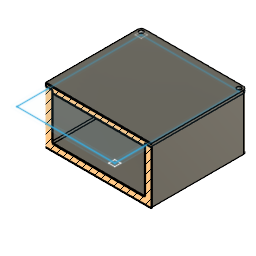
Box (Autodesk Fusion 360 design; units mm, degrees)
part number: 2026-07-20-21-03-58-524
Autodesk Fusion 360 part; units mm, degrees
sketch "Sketch1" plane through (0, 0, 0) normal (0, 0, 1) x (1, 0, 0)
  line L0 (40, -50) -> (-40, -50)
  line L1 (-40, -50) -> (-40, 50)
  line L2 (-40, 50) -> (40, 50)
  line L3 (40, 50) -> (40, -50)
  line L4 (40, -50) -> (-40, 50) construction
  line L5 (-40, -50) -> (40, 50) construction
  dimension "d1" = 80
  dimension "d2" = 100
  constraint horizontal L0
  constraint perpendicular L0 L1
  constraint parallel L0 L2
  constraint parallel L1 L3
  constraint coincident L4 origin
  constraint coincident L5 origin
  measures "d1" distance of L1.end L2.end
  measures "d2" distance of L0.end L1.end
extrude "Extrude1" add sketch "Sketch1" along normal blind 40 makes body 1
shell "Shell1" thickness 5 removed faces 1 at (13.3333, -16.6667, 40) on bodies 1
fillet "Fillet1" radius 2.5 1 edges at (40, -50, 20) on bodies 1
fillet "Fillet2" radius 2.5 1 edges at (40, 50, 20) on bodies 1
fillet "Fillet3" radius 2.5 1 edges at (-40, 50, 20) on bodies 1
fillet "Fillet4" radius 2.5 1 edges at (-40, -50, 20) on bodies 1
fillet "Fillet5" radius 1 8 edges at (-35, -45, 22.5) (0, -45, 5) (-35, 0, 5) (35, -45, 22.5) (35, 0, 5) (35, 45, 22.5) (0, 45, 5) (-35, 45, 22.5) on bodies 1
sketch "Sketch2" plane through (0, 0, 40) normal (0, 0, 1) x (-1, 0, 0)
  arc A0 (40, 47.5) -> (37.5, 50) centre (37.5, 47.5) ccw
  line L0 (37.5, 50) -> (-37.5, 50)
  arc A1 (-37.5, 50) -> (-40, 47.5) centre (-37.5, 47.5) ccw
  line L1 (-40, 47.5) -> (-40, -47.5)
  arc A2 (-40, -47.5) -> (-37.5, -50) centre (-37.5, -47.5) ccw
  line L2 (-37.5, -50) -> (37.5, -50)
  arc A3 (37.5, -50) -> (40, -47.5) centre (37.5, -47.5) ccw
  line L3 (40, -47.5) -> (40, 47.5)
  line L4 (-35, -44) -> (-35, 44)
  arc A4 (-34, 45) -> (-35, 44) centre (-34, 44) ccw
  line L5 (-34, 45) -> (34, 45)
  arc A5 (35, 44) -> (34, 45) centre (34, 44) ccw
  line L6 (35, 44) -> (35, -44)
  arc A6 (34, -45) -> (35, -44) centre (34, -44) ccw
  line L7 (34, -45) -> (-34, -45)
  arc A7 (-35, -44) -> (-34, -45) centre (-34, -44) ccw
  line L8 (-39.2678, 49.2678) -> (-34.7071, 49.2678) construction
  line L9 (-34.7071, 49.2678) -> (-34.7071, 44.7071) construction
  line L10 (-34.7071, 44.7071) -> (-39.2678, 44.7071) construction
  line L11 (-39.2678, 44.7071) -> (-39.2678, 49.2678) construction
  line L12 (34.7071, -44.7071) -> (39.2678, -44.7071) construction
  line L13 (39.2678, -44.7071) -> (39.2678, -49.2678) construction
  line L14 (39.2678, -49.2678) -> (34.7071, -49.2678) construction
  line L15 (34.7071, -49.2678) -> (34.7071, -44.7071) construction
  line L16 (36.9874, -46.9874) -> (-36.9874, -46.9874)
  line L17 (-36.9874, -46.9874) -> (-36.9874, 46.9874)
  line L18 (-36.9874, 46.9874) -> (36.9874, 46.9874)
  line L19 (36.9874, 46.9874) -> (36.9874, -46.9874)
  constraint horizontal L8
  constraint vertical L9
  constraint horizontal L10
  constraint vertical L11
  constraint midpoint A4 L9.end
  constraint midpoint A1 L8.start
  constraint horizontal L12
  constraint vertical L13
  constraint horizontal L14
  constraint vertical L15
  constraint midpoint A3 L13.end
  constraint midpoint A6 L12.start
  constraint horizontal L16
  constraint vertical L17
  constraint horizontal L18
  constraint vertical L19
extrude "Extrude2" add sketch "Sketch2" along normal blind 2 contours A0 L0 A1 L1 A2 L2 A3 L3 | L4 A4 L5 A5 L6 A6 L7 A7 | L16 L17 L18 L19 bodies 1
ref_plane "WorkPlane1" through (0, 0, 40) normal (0, 0, 1) x (-1, 0, 0)
split "Split1" by plane through (0, 0, 40) normal (0, 0, 1) bodies 1 makes body 2 at (13.3333, 15.8333, 42)
sketch "Sketch3" plane through (0, 0, 42) normal (0, 0, 1) x (-1, 0, 0)
  line L0 (40, -47.5) -> (40, 47.5)
  arc A0 (40, 47.5) -> (37.5, 50) centre (37.5, 47.5) ccw
  line L1 (37.5, 50) -> (-37.5, 50)
  arc A1 (-37.5, 50) -> (-40, 47.5) centre (-37.5, 47.5) ccw
  line L2 (-40, 47.5) -> (-40, -47.5)
  arc A2 (-40, -47.5) -> (-37.5, -50) centre (-37.5, -47.5) ccw
  line L3 (-37.5, -50) -> (37.5, -50)
  arc A3 (37.5, -50) -> (40, -47.5) centre (37.5, -47.5) ccw
sketch "Sketch4" plane through (0, 0, 40) normal (0, 0, 1) x (-1, 0, 0)
  line L0 (37, 47) -> (-37, 47) construction
  line L1 (-37, 47) -> (-37, -47) construction
  line L2 (-37, -47) -> (37, -47) construction
  line L3 (37, -47) -> (37, 47) construction
  line L4 (-34, -45) -> (34, -45)
  line L5 (35, -44) -> (35, 44)
  line L6 (34, 45) -> (-34, 45)
  line L7 (-35, 44) -> (-35, -44)
  line L8 (-35, -45) -> (35, 45) construction
  line L9 (35, -45) -> (-35, 45) construction
  arc A0 (35, 44) -> (34, 45) centre (34, 44) ccw
  arc A1 (34, -45) -> (35, -44) centre (34, -44) ccw
  arc A2 (-35, -44) -> (-34, -45) centre (-34, -44) ccw
  arc A3 (-34, 45) -> (-35, 44) centre (-34, 44) ccw
  dimension "d29" = 70
  dimension "d30" = 90
  dimension "d31" = 1
  dimension "d32" = 1
  dimension "d33" = 1
  constraint horizontal L0
  constraint vertical L1
  constraint horizontal L2
  constraint vertical L3
  constraint horizontal L4
  constraint perpendicular L4 L5
  constraint parallel L4 L6
  constraint parallel L5 L7
  constraint coincident L8 origin
  constraint coincident L9 origin
  constraint coincident L8.end L6
  constraint coincident L8.end L5
  constraint tangent L6 A0
  constraint tangent L5 A0
  constraint coincident L9.start L5
  constraint coincident L9.start L4
  constraint tangent L5 A1
  constraint tangent L4 A1
  constraint coincident L8.start L7
  constraint coincident L8.start L4
  constraint tangent L7 A2
  constraint tangent L4 A2
  constraint equal A1 A2
  constraint coincident L9.end L6
  constraint coincident L9.end L7
  constraint tangent L6 A3
  constraint tangent L7 A3
  measures "d29" distance of L8.end L9.end
  measures "d30" distance of L9.start L8.end
  measures "d31" radius of A0
  measures "d32" radius of A1
  measures "d33" radius of A3
hole "Hole5" at (-36.9874, 46.9874, 40) at (36.9874, 46.9874, 40) at (36.9874, -46.9874, 40) at (-36.9874, -46.9874, 40) direction (0, 0, -1) diameter 2.6 depth 7 tip angle 180 bodies 1
extrude "Extrude4" add sketch "Sketch2" against normal blind 2 contours L4 A4 L5 A5 L6 A6 L7 A7 bodies 2
hole "Hole6" at (-36.9874, 46.9874, 40) at (36.9874, 46.9874, 40) at (36.9874, -46.9874, 40) at (-36.9874, -46.9874, 40) direction (0, 0, 1) diameter 3.2 depth 2 tip angle 180 bodies 2
equation "d1 = BoxDepth"
equation "d2 = BoxWidth"
equation "BoxWidth = 100 mm"
equation "BoxDepth = 80 mm"
equation "BoxHeight = 40 mm"
equation "WallThickness = 5 mm"
equation "d9 = WallThickness"
equation "OuterFillet = 2.5 mm"
equation "d12 = OuterFillet"
equation "d14 = OuterFillet"
equation "d16 = OuterFillet"
equation "d18 = OuterFillet"
equation "InnerFillet = 1 mm"
equation "d21 = InnerFillet"
equation "d31 = InnerFillet"
equation "d32 = InnerFillet"
equation "d33 = InnerFillet"
